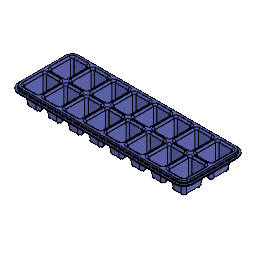
Ice Cube Tray (Autodesk Fusion 360 design; units mm, degrees)
Autodesk Fusion 360 part; units mm, degrees
sketch "Sketch1" plane through (0, 0, 0) normal (0, 0, 1) x (1, 0, 0)
  line L0 (152.4, 50.8) -> (-152.4, 50.8)
  line L1 (-152.4, 50.8) -> (-152.4, -50.8)
  line L2 (-152.4, -50.8) -> (152.4, -50.8)
  line L3 (152.4, -50.8) -> (152.4, 50.8)
  line L4 (152.4, 50.8) -> (-152.4, -50.8) construction
  line L5 (-152.4, 50.8) -> (152.4, -50.8) construction
  dimension "d1" = 304.8
  dimension "d2" = 101.6
  constraint perpendicular L0 L1
  constraint parallel L0 L2
  constraint parallel L1 L3
  constraint horizontal L0
  constraint coincident L4 origin
  constraint coincident L5 origin
  measures "d1" distance of L1.end L2.end
  measures "d2" distance of L0.end L1.end
extrude "Extrude1" add sketch "Sketch1" along normal blind 50.8
sketch "Sketch2" plane through (0, 0, 50.8) normal (0, 0, 1) x (-1, 0, 0)
  line L0 (-152.4, 50.8) -> (-152.4, -50.8)
  line L1 (-152.4, -50.8) -> (152.4, -50.8)
  line L2 (152.4, -50.8) -> (152.4, 50.8)
  line L3 (152.4, 50.8) -> (-152.4, 50.8)
  line L4 (147.32, 45.72) -> (116.84, 45.72)
  line L5 (116.84, 45.72) -> (116.84, 3.81)
  line L6 (116.84, 3.81) -> (147.32, 3.81)
  line L7 (147.32, 3.81) -> (147.32, 45.72)
  dimension "d5" = 30.48
  dimension "d6" = 41.91
  dimension "d7" = 5.08
  dimension "d8" = 5.08
  constraint horizontal L4
  constraint vertical L5
  constraint horizontal L6
  constraint vertical L7
  measures "d5" distance of L4.start L4.end
  measures "d6" distance of L4.start L6.end
  measures "d7" distance of L2 L7
  measures "d8" distance of L3 L4
extrude "Extrude2" cut sketch "Sketch2" against normal blind 33.02 draft -10 contours L4 L5 L6 L7
fillet "Fillet1" radius 3.302 12 edges at (-116.84, -24.765, 50.8) (-119.7512, -6.7212, 34.29) (-132.08, -3.81, 50.8) (-144.4088, -6.7212, 34.29) (-147.32, -24.765, 50.8) (-144.4088, -42.8088, 34.29) (-132.08, -45.72, 50.8) (-119.7512, -42.8088, 34.29) (-122.6623, -24.765, 17.78) (-132.08, -9.6323, 17.78) (-141.4977, -24.765, 17.78) (-132.08, -39.8977, 17.78)
pattern_linear "R-Pattern1" count 8 spacing 37.7371 along (1, 0, 0) count 2 spacing 49.53 along (0, 1, 0) of "Extrude2", "Fillet1"
shell "Shell1" thickness 1.778 removed faces 5 at (50.8, -50.8, 33.8667) at (-152.4, 16.9333, 33.8667) at (-50.8, 50.8, 33.8667) at (152.4, -16.9333, 33.8667) at (-50.8, 16.9333, 0)
fillet "Fillet2" radius 10.16 4 edges at (-152.4, 50.8, 49.911) (-152.4, -50.8, 49.911) (152.4, -50.8, 49.911) (152.4, 50.8, 49.911)
sketch "Sketch3" plane through (0, 0, 0) normal (0, 1, 0) x (1, 0, 0)
  line L0 (152.4, -50.8) -> (152.4, -46.99)
  line L1 (154.94, -44.45) -> (158.75, -44.45)
  line L2 (158.75, -44.45) -> (158.75, -46.228)
  line L3 (152.4, -50.8) -> (154.178, -50.8)
  line L4 (158.75, -46.228) -> (155.448, -46.228)
  line L5 (154.178, -47.498) -> (154.178, -50.8)
  arc A0 (154.94, -44.45) -> (152.4, -46.99) centre (154.94, -46.99) ccw
  arc A1 (155.448, -46.228) -> (154.178, -47.498) centre (155.448, -47.498) ccw
  point P0 (152.4, -44.45)
  dimension "d18" = 6.35
  dimension "d19" = 6.35
  dimension "d21" = 1.778
  dimension "d23" = 2.54
  dimension "d24" = 1.27
  constraint vertical L0
  constraint perpendicular L0 L1
  constraint perpendicular L1 L2
  constraint perpendicular L0 L3
  constraint perpendicular L2 L4
  constraint perpendicular L4 L5
  constraint coincident P0 L0
  constraint coincident P0 L1
  constraint tangent L0 A0
  constraint tangent L1 A0
  constraint tangent L5 A1
  constraint tangent L4 A1
  measures "d18" distance of L0.start P0
  measures "d19" distance of P0 L1.end
  measures "d21" distance of L0.start L3.end
  measures "d23" radius of A0
  measures "d24" radius of A1
sweep "Sweep1" add profiles "Sketch3" along 8 edges at (-149.4242, 47.8242, 50.8) (-152.4, 0, 50.8) (-149.4242, -47.8242, 50.8) (0, -50.8, 50.8) (149.4242, -47.8242, 50.8) (152.4, 0, 50.8) (149.4242, 47.8242, 50.8) (0, 50.8, 50.8) section 1
